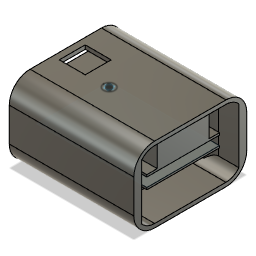
20201123 v1 (Autodesk Fusion 360 design; units mm, degrees)
Autodesk Fusion 360 part; units mm, degrees
note: some values were not read from the file. Chosen so that the rebuilt part matches the saved one: which bodies a step acts on; which face or edge a step refers to.
sketch "Sketch1" plane through (0, 0, 0) normal (0, 1, 0) x (1, 0, 0)
  line L0 (-42.5, 28) -> (42.5, 28)
  line L1 (42.5, 28) -> (42.5, -28)
  line L2 (42.5, -28) -> (-42.5, -28)
  line L3 (-42.5, -28) -> (-42.5, 28)
  line L4 (-42.5, 28) -> (42.5, -28) construction
  line L5 (42.5, 28) -> (-42.5, -28) construction
  line L6 (-42.5, 28) -> (-39, 28) construction
  line L7 (-39, 28) -> (-39, 24.5) construction
  line L8 (-39, 24.5) -> (-42.5, 24.5) construction
  line L9 (-42.5, 24.5) -> (-42.5, 28) construction
  line L10 (-39, 24.5) -> (19, 24.5) construction
  line L11 (19, 24.5) -> (19, -24.5) construction
  line L12 (19, -24.5) -> (-39, -24.5) construction
  line L13 (-39, -24.5) -> (-39, 24.5) construction
  circle A0 centre (-39, 24.5) radius 1.25
  circle A1 centre (19, 24.5) radius 1.25
  circle A2 centre (-39, -24.5) radius 1.25
  circle A3 centre (19, -24.5) radius 1.25
  dimension "d1" = 85
  dimension "d2" = 56
  dimension "d3" = 3.5
  dimension "d4" = 3.5
  dimension "d5" = 58
  dimension "d6" = 49
  dimension "d7" = 2.5
  dimension "d10" = 58
  dimension "d11" = -49
  constraint horizontal L0
  constraint perpendicular L0 L1
  constraint parallel L0 L2
  constraint parallel L1 L3
  constraint coincident L4 origin
  constraint coincident L5 origin
  constraint horizontal L6
  constraint vertical L7
  constraint horizontal L8
  constraint vertical L9
  constraint horizontal L10
  constraint vertical L11
  constraint horizontal L12
  constraint vertical L13
  constraint coincident L7.end L8.start
  measures "d1" distance of L1.end L2.end
  measures "d2" distance of L0.end L1.end
  measures "d3" distance of L0.start L6.end
  measures "d4" distance of L0.start L8.end
  measures "d5" distance of L7.end L10.end
  measures "d6" distance of L7.end L12.end
  measures "d7" diameter of A0
extrude "Extrude1" add sketch "Sketch1" along normal blind 1.5 makes body 1
sketch "Sketch2" plane through (0, 1.5, 0) normal (0, 1, 0) x (-1, 0, 0)
  circle A0 centre (-19, -24.5) radius 1.25
  circle A1 centre (39, 24.5) radius 1.25
  circle A2 centre (-19, 24.5) radius 1.25
  circle A3 centre (39, -24.5) radius 1.25
  line L0 (42.5, 28) -> (-42.5, 28)
  line L1 (-42.5, 28) -> (-42.5, -28)
  line L2 (-42.5, -28) -> (42.5, -28)
  line L3 (42.5, -28) -> (42.5, 28)
  line L4 (40.3568, -26.85) -> (41.7135, -24.5)
  line L5 (41.7135, -24.5) -> (40.3568, -22.15)
  line L6 (40.3568, -22.15) -> (37.6432, -22.15)
  line L7 (37.6432, -22.15) -> (36.2865, -24.5)
  line L8 (36.2865, -24.5) -> (37.6432, -26.85)
  line L9 (37.6432, -26.85) -> (40.3568, -26.85)
  circle A4 centre (39, -24.5) radius 4.25
  point P0 (39, -24.5)
  dimension "d14" = 2.35
  dimension "d15" = 8.5
  constraint coincident P0 A3.centre
  constraint concentric A3 A4
  measures "d14" distance of P0 L9
  measures "d15" diameter of A4
extrude "Extrude2" add sketch "Sketch2" along normal blind 5 separate body contours L3 A4 | L2 L3 A4 | L2 A4 picked at (36.4205, -25.9987) makes body 2
move_body "Move1" bodies 2 to x (1, 0, 0) y (0, 1, 0) z (0, 0, 1) at (0, 2, 0)
copy_body "Body->Comp1" bodies 1 removing the originals makes body 3 in component "raspberry"
copy_body "CutPasteBodies1" bodies 2 removing the originals makes body 4 in component "raspberry"
pattern_linear "R-Pattern1" count 2 spacing 58 along (1, 0, 0) count 2 spacing 49 along (0, 0, 1) of bodies 4 makes body 5 at (21.5784, 6.8333, -27.8785) makes body 6 at (-36.4216, 6.8333, 21.1215) makes body 7 at (21.5784, 6.8333, 21.1215) in component "raspberry"
copy_body "CopyPasteBodies1" bodies 3 makes body 8
move_body "Move2" bodies 8 to x (1, 0, 0) y (0, 1, 0) z (0, 0, 1) at (0, 9, 0)
move_body "Move3" bodies 8 to x (1, 0, 0) y (0, 1, 0) z (0, 0, 1) at (0, -0.5, 0)
extrude "Extrude1'" add 1 faces at (-19.3123, 0, 7.8904) along direction (0, -1, 0) blind 16 on bodies 3 bodies 3 in component "raspberry"
extrude "Extrude3" add 1 faces at (-19.3123, 10, 7.8904) along direction (0, 1, 0) blind 0.15 on bodies 8 bodies 8
extrude "Extrude4" cut 1 faces at (-19.3123, 10.15, 7.8904) along direction (0, -1, 0) blind 0.03 on bodies 8 bodies 8
sketch "Sketch3" plane through (0, 10.12, 0) normal (0, 1, 0) x (-1, 0, 0)
  circle A0 centre (-19, -24.5) radius 1.25
  circle A1 centre (39, 24.5) radius 1.25
  circle A2 centre (-19, 24.5) radius 1.25
  circle A3 centre (39, -24.5) radius 1.25
  line L0 (42.5, 28) -> (-42.5, 28)
  line L1 (-42.5, 28) -> (-42.5, -28)
  line L2 (-42.5, -28) -> (42.5, -28)
  line L3 (42.5, -28) -> (42.5, 28)
  line L4 (-42.5, 20) -> (42.5, 20)
  line L5 (42.5, 20) -> (42.5, -20)
  line L6 (42.5, -20) -> (-42.5, -20)
  line L7 (-42.5, -20) -> (-42.5, 20)
  line L8 (-42.5, 20) -> (42.5, -20) construction
  line L9 (42.5, 20) -> (-42.5, -20) construction
  dimension "d28" = 40
  constraint horizontal L4
  constraint perpendicular L4 L5
  constraint parallel L4 L6
  constraint parallel L5 L7
  constraint coincident L8 origin
  constraint coincident L9 origin
  measures "d28" distance of L4.end L5.end
extrude "Extrude5" add sketch "Sketch3" along normal blind 20 contours L1 L3 L4 L5 L6 L7 bodies 8
sketch "Sketch4" plane through (0, 3.5, 0) normal (0, -1, 0) x (1, 0, 0)
  line L0 (-37.6432, 22.15) -> (-40.3568, 22.15)
  line L1 (-40.3568, 22.15) -> (-41.7135, 24.5)
  line L2 (-41.7135, 24.5) -> (-40.3568, 26.85)
  line L3 (-40.3568, 26.85) -> (-37.6432, 26.85)
  line L4 (-37.6432, 26.85) -> (-36.2865, 24.5)
  line L5 (-36.2865, 24.5) -> (-37.6432, 22.15)
  circle A0 centre (-39, 24.5) radius 4.25
  line L6 (45, 28.5) -> (45, -28.5)
  line L7 (-45, -23.5) -> (-45, 23.5)
  line L8 (45, 37.5) -> (-45, -37.5) construction
  line L9 (-34.75, 24.5) -> (-34.75, 28.5)
  line L10 (-45, 0) -> (45, 0) construction
  line L11 (19, 37) -> (-39, 37) construction
  line L12 (-10, 37) -> (-10, -37.5) construction
  line L13 (23.25, 24.5) -> (23.25, 28.5)
  line L14 (14.75, 24.5) -> (14.75, 28.5)
  circle A1 centre (19, 24.5) radius 4.25
  circle A2 centre (-39, 24.5) radius 4.25
  line L15 (23.25, -24.5) -> (23.25, -28.5)
  line L16 (14.75, -24.5) -> (14.75, -28.5)
  circle A3 centre (19, -24.5) radius 4.25
  line L17 (-34.75, -24.5) -> (-34.75, -28.5)
  circle A4 centre (-39, -24.5) radius 4.25
  line L18 (48, -40.5) -> (-48, -40.5)
  line L19 (-48, -40.5) -> (-48, 40.5)
  line L20 (-48, 40.5) -> (48, 40.5)
  line L21 (48, 40.5) -> (48, -40.5)
  line L22 (32.25, 37.5) -> (36, 37.5)
  line L23 (-45, 37.5) -> (-10, 8.3333) construction
  line L24 (0, 0) -> (45, -37.5) construction
  line L25 (-25.75, 37.5) -> (5.75, 37.5)
  line L26 (36, -37.5) -> (32.25, -37.5)
  line L27 (5.75, -37.5) -> (-25.75, -37.5)
  line L28 (-43.25, -24.5) -> (-44, -24.5)
  line L29 (-43.25, 24.5) -> (-44, 24.5)
  arc A5 (5.75, -37.5) -> (14.75, -28.5) centre (5.75, -28.5) ccw
  arc A6 (23.25, -28.5) -> (32.25, -37.5) centre (32.25, -28.5) ccw
  arc A7 (32.25, 37.5) -> (23.25, 28.5) centre (32.25, 28.5) ccw
  arc A8 (14.75, 28.5) -> (5.75, 37.5) centre (5.75, 28.5) ccw
  arc A9 (-25.75, 37.5) -> (-34.75, 28.5) centre (-25.75, 28.5) ccw
  arc A10 (-34.75, -28.5) -> (-25.75, -37.5) centre (-25.75, -28.5) ccw
  arc A11 (36, -37.5) -> (45, -28.5) centre (36, -28.5) ccw
  arc A12 (45, 28.5) -> (36, 37.5) centre (36, 28.5) ccw
  arc A13 (-44, 24.5) -> (-45, 23.5) centre (-44, 23.5) ccw
  arc A14 (-45, -23.5) -> (-44, -24.5) centre (-44, -23.5) ccw
  dimension "d31" = 90
  dimension "d32" = 75
  dimension "d34" = 9
  dimension "d35" = 1
  constraint parallel L6 L7
  constraint coincident L24.start L23
  constraint coincident L8 L24.start
  constraint coincident L24.start origin
  constraint coincident A0 L29.start
  constraint coincident A0 L9.start
  constraint tangent A0 L9
  constraint parallel L3 L11
  constraint midpoint L11 L12.start
  constraint coincident L12.end L26
  constraint perpendicular L12 L26
  constraint symmetric L29.start L12 L13.start
  constraint symmetric L9.start L12 L14.start
  constraint coincident L14.start A1
  constraint tangent L14 A1
  constraint coincident L13.start A1
  constraint coincident L29.start A2
  constraint coincident L9.start A2
  constraint symmetric L29.start L10 L28.start
  constraint symmetric L9.start L10 L17.start
  constraint symmetric L10 L13.start L15.start
  constraint symmetric L10 L14.start L16.start
  constraint symmetric L10 A1 A3
  constraint symmetric L10 A2 A4
  constraint parallel L18 L26
  constraint parallel L7 L19
  constraint parallel L6 L21
  constraint coincident L12 L23.end
  constraint collinear L23 L24
  constraint collinear L26 L27
  constraint perpendicular L7 L29
  constraint coincident L7 L10.start
  constraint tangent L16 A5
  constraint tangent L27 A5
  constraint tangent L15 A6
  constraint tangent L26 A6
  constraint equal A5 A6
  constraint tangent L13 A7
  constraint tangent L22 A7
  constraint equal A5 A7
  constraint tangent L14 A8
  constraint tangent L25 A8
  constraint equal A5 A8
  constraint tangent L9 A9
  constraint tangent L25 A9
  constraint equal A5 A9
  constraint tangent L17 A10
  constraint tangent L27 A10
  constraint equal A5 A10
  constraint coincident L6 L10.end
  constraint coincident L24.end L26
  constraint coincident L24.end L6
  constraint tangent L26 A11
  constraint tangent L6 A11
  constraint equal A5 A11
  constraint coincident L8.start L6
  constraint coincident L8.start L22
  constraint tangent L6 A12
  constraint tangent L22 A12
  constraint equal A5 A12
  constraint tangent L29 A13
  constraint tangent L7 A13
  constraint tangent L28 A14
  constraint tangent L7 A14
  constraint equal A13 A14
  measures "d31" distance of L24.end L8.end
  measures "d32" distance of L8.start L24.end
  measures "d34" radius of A5
  measures "d35" radius of A13
extrude "Extrude2'" add sketch "Sketch4" against normal blind 5 contours L18 L19 L20 L21 bodies 4 5 6 7 in component "raspberry"
copy_body "CutPasteBodies2" bodies 8 removing the originals makes body 9 in component "raspberry"
copy_body "CopyPasteBodies2" bodies 4 makes body 10
move_body "Move4" bodies 10 to x (1, 0, 0) y (0, 1, 0) z (0, 0, 1) at (0, 6.5, 0)
move_body "Move5" bodies 10 to x (1, 0, 0) y (0, 1, 0) z (0, 0, 1) at (0, 10, 0)
move_body "Move6" bodies 10 to x (1, 0, 0) y (0, 1, 0) z (0, 0, 1) at (0, -9.88, 0)
extrude "Extrude6" cut 1 faces at (-40.7645, 15.12, -33.1962) along direction (0, -1, 0) blind 2 on bodies 10 bodies 10
sketch "Sketch5" plane through (0, 8.5, 0) normal (0, 1, 0) x (-1, 0, 0)
  line L0 (-17.6432, 22.15) -> (-20.3568, 22.15)
  line L1 (-20.3568, 22.15) -> (-21.7135, 24.5)
  line L2 (-21.7135, 24.5) -> (-20.3568, 26.85)
  line L3 (-20.3568, 26.85) -> (-17.6432, 26.85)
  line L4 (-17.6432, 26.85) -> (-16.2865, 24.5)
  line L5 (-16.2865, 24.5) -> (-17.6432, 22.15)
  line L6 (40.3568, 22.15) -> (37.6432, 22.15)
  line L7 (37.6432, 22.15) -> (36.2865, 24.5)
  line L8 (36.2865, 24.5) -> (37.6432, 26.85)
  line L9 (37.6432, 26.85) -> (40.3568, 26.85)
  line L10 (40.3568, 26.85) -> (41.7135, 24.5)
  line L11 (41.7135, 24.5) -> (40.3568, 22.15)
  line L12 (-17.6432, -26.85) -> (-20.3568, -26.85)
  line L13 (-20.3568, -26.85) -> (-21.7135, -24.5)
  line L14 (-21.7135, -24.5) -> (-20.3568, -22.15)
  line L15 (-20.3568, -22.15) -> (-17.6432, -22.15)
  line L16 (-17.6432, -22.15) -> (-16.2865, -24.5)
  line L17 (-16.2865, -24.5) -> (-17.6432, -26.85)
  line L18 (48, 40.5) -> (-48, 40.5)
  line L19 (-48, 40.5) -> (-48, -40.5)
  line L20 (-48, -40.5) -> (48, -40.5)
  line L21 (48, -40.5) -> (48, 40.5)
  line L22 (40.3568, -26.85) -> (37.6432, -26.85)
  line L23 (37.6432, -26.85) -> (36.2865, -24.5)
  line L24 (36.2865, -24.5) -> (37.6432, -22.15)
  line L25 (37.6432, -22.15) -> (40.3568, -22.15)
  line L26 (40.3568, -22.15) -> (41.7135, -24.5)
  line L27 (41.7135, -24.5) -> (40.3568, -26.85)
  arc A0 (43.25, -24.5) -> (34.75, -24.5) centre (39, -24.5) ccw
  line L28 (34.75, -24.5) -> (34.75, -28.5)
  arc A1 (25.75, -37.5) -> (34.75, -28.5) centre (25.75, -28.5) ccw
  line L29 (25.75, -37.5) -> (-5.75, -37.5)
  arc A2 (-14.75, -28.5) -> (-5.75, -37.5) centre (-5.75, -28.5) ccw
  line L30 (-14.75, -28.5) -> (-14.75, -24.5)
  arc A3 (-14.75, -24.5) -> (-23.25, -24.5) centre (-19, -24.5) ccw
  line L31 (-23.25, -24.5) -> (-23.25, -28.5)
  arc A4 (-32.25, -37.5) -> (-23.25, -28.5) centre (-32.25, -28.5) ccw
  line L32 (-32.25, -37.5) -> (-36, -37.5)
  arc A5 (-45, -28.5) -> (-36, -37.5) centre (-36, -28.5) ccw
  line L33 (-45, -28.5) -> (-45, 28.5)
  arc A6 (-36, 37.5) -> (-45, 28.5) centre (-36, 28.5) ccw
  line L34 (-36, 37.5) -> (-32.25, 37.5)
  arc A7 (-23.25, 28.5) -> (-32.25, 37.5) centre (-32.25, 28.5) ccw
  line L35 (-23.25, 28.5) -> (-23.25, 24.5)
  arc A8 (-23.25, 24.5) -> (-14.75, 24.5) centre (-19, 24.5) ccw
  line L36 (-14.75, 24.5) -> (-14.75, 28.5)
  arc A9 (-5.75, 37.5) -> (-14.75, 28.5) centre (-5.75, 28.5) ccw
  line L37 (-5.75, 37.5) -> (25.75, 37.5)
  arc A10 (34.75, 28.5) -> (25.75, 37.5) centre (25.75, 28.5) ccw
  line L38 (34.75, 28.5) -> (34.75, 24.5)
  arc A11 (34.75, 24.5) -> (43.25, 24.5) centre (39, 24.5) ccw
  line L39 (43.25, 24.5) -> (44, 24.5)
  arc A12 (45, 23.5) -> (44, 24.5) centre (44, 23.5) ccw
  line L40 (45, 23.5) -> (45, -23.5)
  arc A13 (44, -24.5) -> (45, -23.5) centre (44, -23.5) ccw
  line L41 (44, -24.5) -> (43.25, -24.5)
  line L42 (-19, 24.5) -> (-19, 28.25) construction
  line L43 (39, 24.5) -> (39, 28.25) construction
  arc A14 (48, 36.4333) -> (43.25, 28.5) centre (52.25, 28.5) ccw construction
  line L44 (43.25, 28.5) -> (43.25, 24.5)
  arc A15 (48, 36.4333) -> (43.25, 28.5) centre (52.25, 28.5) ccw
  line L45 (-36, 37.5) -> (-48, 37.5)
  line L46 (48, 28.25) -> (-48, 28.25) construction
  line L47 (-48, 28.25) -> (-48, -28.25) construction
  line L48 (-48, -28.25) -> (48, -28.25) construction
  line L49 (48, -28.25) -> (48, 28.25) construction
  line L50 (48, 28.25) -> (-48, -28.25) construction
  line L51 (-48, 28.25) -> (48, -28.25) construction
  line L52 (-48, 28.25) -> (48, 28.25)
  line L53 (48, -28.25) -> (-48, -28.25)
  line L54 (-48, 0) -> (48, 0) construction
  arc A16 (43.25, -28.5) -> (48, -36.4333) centre (52.25, -28.5) ccw construction
  arc A17 (43.25, -28.5) -> (48, -36.4333) centre (52.25, -28.5) ccw
  line L55 (43.25, -28.5) -> (43.25, -24.5)
  line L56 (-36, -37.5) -> (-48, -37.5)
  dimension "d40" = 3.75
  dimension "d41" = 3.75
  dimension "d42" = 9
  constraint coincident A8.centre L42.start
  constraint vertical L42
  constraint coincident A11.centre L43.start
  constraint parallel L38 L43
  constraint coincident A11.end L39.start
  constraint concentric A14 A15
  constraint coincident L21 A14.start
  constraint coincident A6.start L34.start
  constraint coincident L19 L45.end
  constraint tangent A6 L45
  constraint horizontal L46
  constraint perpendicular L46 L47
  constraint parallel L46 L48
  constraint parallel L47 L49
  constraint coincident L21 L46.start
  constraint coincident L50 origin
  constraint coincident L51 origin
  constraint midpoint L19 L54.start
  constraint midpoint L21 L54.end
  constraint symmetric A11.end L54 A0.start
  constraint symmetric A14.end L54 A16.start
  constraint symmetric A14 L54 A16
  constraint symmetric A15 L54 A17
  constraint symmetric A14.start L54 A16.end
  constraint coincident L32.end A5.end
  constraint coincident L19 L56.end
  constraint tangent A5 L56
  measures "d40" distance of A8.centre L42.end
  measures "d41" distance of A11.centre L43.end
  measures "d42" radius of A14
extrude "Extrude3'" cut sketch "Sketch5" against normal blind 25 contours L21 L44 A15 L52 | L19 L33 A6 L45 L52 | L21 L39 A12 L40 A13 L41 L44 L52 L53 L55 | L19 L33 L52 L53 | L21 L53 A17 L55 | L19 A5 L33 L53 L56 bodies 4 makes body 11 at (-41.9239, 8.5, 36.3378) in component "raspberry"
extrude "Extrude7" add sketch "Sketch5" along normal blind 2 contours L19 L20 L21 L28 A1 L29 A2 L30 L31 A4 L32 L53 A17 L55 L56 bodies 10
extrude "Extrude8" add sketch "Sketch5" along normal blind 3 contours L18 L19 L21 L34 A7 L35 L36 A9 L37 A10 L38 L44 A15 L45 L52 bodies 10
extrude "Extrude9" cut sketch "Sketch5" along normal blind 20 contours L21 L44 A15 L52 | L19 L33 A6 L45 L52 | L21 L39 A12 L40 A13 L41 L44 L52 L53 L55 | L19 L33 L52 L53 | L21 L53 A17 L55 | L19 A5 L33 L53 L56 bodies 10 makes body 12 at (-41.9239, 13.12, 36.3378)
combine "Combine1" operation add target body 10 tool bodies 4
combine "Combine2" operation add target body 12 tool bodies 11
copy_body "CutPasteBodies3" bodies 12 removing the originals makes body 13 in component "raspberry"
copy_body "CutPasteBodies4" bodies 10 removing the originals makes body 14 in component "raspberry"
sketch "Sketch6" plane through (0, 13.12, 0) normal (0, 1, 0) x (-1, 0, 0)
  line L0 (40.3568, -26.85) -> (37.6432, -26.85)
  line L1 (37.6432, -26.85) -> (36.2865, -24.5)
  line L2 (36.2865, -24.5) -> (37.6432, -22.15)
  line L3 (37.6432, -22.15) -> (40.3568, -22.15)
  line L4 (40.3568, -22.15) -> (41.7135, -24.5)
  line L5 (41.7135, -24.5) -> (40.3568, -26.85)
  line L6 (-17.6432, -26.85) -> (-20.3568, -26.85)
  line L7 (-20.3568, -26.85) -> (-21.7135, -24.5)
  line L8 (-21.7135, -24.5) -> (-20.3568, -22.15)
  line L9 (-20.3568, -22.15) -> (-17.6432, -22.15)
  line L10 (-17.6432, -22.15) -> (-16.2865, -24.5)
  line L11 (-16.2865, -24.5) -> (-17.6432, -26.85)
  line L12 (-32.25, -37.5) -> (-48, -37.5)
  line L13 (-48, -37.5) -> (-48, -40.5)
  line L14 (-48, -40.5) -> (48, -40.5)
  line L15 (48, -40.5) -> (48, -36.4333)
  arc A0 (43.25, -28.5) -> (48, -36.4333) centre (52.25, -28.5) ccw
  line L16 (43.25, -28.5) -> (43.25, -24.5)
  arc A1 (43.25, -24.5) -> (34.75, -24.5) centre (39, -24.5) ccw
  line L17 (34.75, -24.5) -> (34.75, -28.5)
  arc A2 (25.75, -37.5) -> (34.75, -28.5) centre (25.75, -28.5) ccw
  line L18 (25.75, -37.5) -> (-5.75, -37.5)
  arc A3 (-14.75, -28.5) -> (-5.75, -37.5) centre (-5.75, -28.5) ccw
  line L19 (-14.75, -28.5) -> (-14.75, -24.5)
  arc A4 (-14.75, -24.5) -> (-23.25, -24.5) centre (-19, -24.5) ccw
  line L20 (-23.25, -24.5) -> (-23.25, -28.5)
  arc A5 (-32.25, -37.5) -> (-23.25, -28.5) centre (-32.25, -28.5) ccw
  circle A6 centre (-19, -24.5) radius 1.375
  circle A7 centre (-19, -24.5) radius 2.7135
  circle A8 centre (39, -24.5) radius 2.7135
  circle A9 centre (39, -24.5) radius 1.375
  circle A10 centre (-19, 24.5) radius 2.7135
  circle A11 centre (-19, 24.5) radius 1.375
  circle A12 centre (39, 24.5) radius 2.7135
  circle A13 centre (39, 24.5) radius 1.375
  dimension "d51" = 2.75
  dimension "d54" = 58
  dimension "d55" = 49
  constraint concentric A4 A6
  constraint concentric A6 A7
  constraint coincident L6.start A7
  measures "d51" diameter of A6
extrude "Extrude5'" add sketch "Sketch6" against normal blind 3 contours L0 L1 L2 L3 L4 L5 | L6 L7 L8 L9 L10 L11 | A10 | A12 bodies 13 14 in component "raspberry"
extrude "Extrude4'" cut sketch "Sketch6" against normal blind 3 contours L0 L1 L2 L3 L4 L5 | L6 L7 L8 L9 L10 L11 | A10 | A12 bodies 13 in component "raspberry"
extrude "Extrude6'" add sketch "Sketch6" against normal blind 3 contours A10 | A12 bodies 13 in component "raspberry"
extrude "Extrude7'" cut 1 faces at (-19.3123, -16, 7.8904) along direction (0, 1, 0) blind 16 on bodies 3 bodies 3 in component "raspberry"
extrude "Extrude10" add sketch "Sketch2" along normal blind 7 separate body contours L4 L5 L6 L7 L8 L9 makes body 15
copy_body "CopyPasteBodies3" bodies 15 makes body 16
move_body "Move7" bodies 16 to x (1, 0, 0) y (0, 1, 0) z (0, 0, 1) at (0, -18, 0)
move_body "Move8" bodies 16 to x (1, 0, 0) y (0, 1, 0) z (0, 0, 1) at (0, 9.5, 0)
pattern_linear "R-Pattern1'" count 2 spacing 49 along (0, 0, 1) count 2 spacing 58 along (1, 0, 0) of bodies 16 15 makes body 17 at (-40.2438, 6.1667, 24.3755) makes body 18 at (17.7562, 6.1667, -24.6245) makes body 19 at (17.7562, 6.1667, 24.3755) makes body 20 at (-40.2438, -2.3333, 24.3755) makes body 21 at (17.7562, -2.3333, -24.6245) makes body 22 at (17.7562, -2.3333, 24.3755)
copy_body "CopyPasteBodies4" bodies 3 makes body 23
move_body "Move9" bodies 23 to x (1, 0, 0) y (0, 1, 0) z (0, 0, 1) at (0, -40, 0)
move_body "Move10" bodies 23 to x (1, 0, 0) y (0, 1, 0) z (0, 0, 1) at (0, 31.5, 0)
extrude "Extrude11" cut 1 faces at (42.5, -8, -9.3333) along direction (-1, 0, 0) blind 19 on bodies 23 bodies 23
extrude "Extrude12" add 1 faces at (-19.3612, -8.5, 7.8833) along direction (0, -1, 0) blind 8.6 on bodies 23 bodies 23
sketch "Sketch7" plane through (-48, 0, 0) normal (-1, 0, 0) x (0, 0, 1)
  line L0 (-36.4333, 3.5) -> (-36.4333, 13.12)
  line L1 (-36.4333, 13.12) -> (-40.5, 13.12)
  line L2 (-40.5, 13.12) -> (-40.5, 3.5)
  line L3 (-40.5, 3.5) -> (-36.4333, 3.5)
  line L4 (-27.5, 32) -> (27.5, 32)
  line L5 (40.5, 19) -> (40.5, -7)
  line L6 (27.5, -20) -> (-27.5, -20)
  line L7 (-40.5, -7) -> (-40.5, 19)
  line L8 (-40.5, 32) -> (40.5, -20) construction
  line L9 (40.5, 32) -> (-40.5, -20) construction
  arc A0 (-27.5, 32) -> (-40.5, 19) centre (-27.5, 19) ccw
  arc A1 (-40.5, -7) -> (-27.5, -20) centre (-27.5, -7) ccw
  arc A2 (27.5, -20) -> (40.5, -7) centre (27.5, -7) ccw
  arc A3 (40.5, 19) -> (27.5, 32) centre (27.5, 19) ccw
  arc A4 (43.5, 19) -> (27.5, 35) centre (27.5, 19) ccw
  line L10 (-27.5, 35) -> (27.5, 35)
  arc A5 (-27.5, 35) -> (-43.5, 19) centre (-27.5, 19) ccw
  line L11 (-43.5, -7) -> (-43.5, 19)
  arc A6 (-43.5, -7) -> (-27.5, -23) centre (-27.5, -7) ccw
  line L12 (27.5, -23) -> (-27.5, -23)
  arc A7 (27.5, -23) -> (43.5, -7) centre (27.5, -7) ccw
  line L13 (43.5, 19) -> (43.5, -7)
  point P0 (0, 6)
  dimension "d74" = 52
  dimension "d75" = 13
  dimension "d76" = -3
  constraint horizontal L4
  constraint perpendicular L4 L5
  constraint parallel L4 L6
  constraint parallel L5 L7
  constraint coincident L8 P0
  constraint coincident L9 P0
  constraint coincident L8.start L4
  constraint coincident L8.start L7
  constraint tangent L4 A0
  constraint tangent L7 A0
  constraint coincident L9.end L7
  constraint coincident L9.end L6
  constraint tangent L7 A1
  constraint tangent L6 A1
  constraint equal A0 A1
  constraint coincident L8.end L6
  constraint coincident L8.end L5
  constraint tangent L6 A2
  constraint tangent L5 A2
  constraint equal A0 A2
  constraint coincident L9.start L5
  constraint coincident L9.start L4
  constraint tangent L5 A3
  constraint tangent L4 A3
  constraint equal A0 A3
  measures "d74" distance of L9.start L8.end
  measures "d75" radius of A0
extrude "Extrude8'" add sketch "Sketch7" against normal blind 96 bodies 13 14 in component "raspberry"
sketch "Sketch8" plane through (0, 13.12, 0) normal (0, 1, 0) x (-1, 0, 0)
  circle A0 centre (-19, -24.5) radius 1.375
  circle A1 centre (39, -24.5) radius 1.375
  line L0 (-32.25, -37.5) -> (-48, -37.5)
  line L1 (-48, -37.5) -> (-48, -40.5)
  line L2 (-48, -40.5) -> (48, -40.5)
  line L3 (48, -40.5) -> (48, -36.4333)
  arc A2 (43.25, -28.5) -> (48, -36.4333) centre (52.25, -28.5) ccw
  line L4 (43.25, -28.5) -> (43.25, -24.5)
  arc A3 (43.25, -24.5) -> (34.75, -24.5) centre (39, -24.5) ccw
  line L5 (34.75, -24.5) -> (34.75, -28.5)
  arc A4 (25.75, -37.5) -> (34.75, -28.5) centre (25.75, -28.5) ccw
  line L6 (25.75, -37.5) -> (-5.75, -37.5)
  arc A5 (-14.75, -28.5) -> (-5.75, -37.5) centre (-5.75, -28.5) ccw
  line L7 (-14.75, -28.5) -> (-14.75, -24.5)
  arc A6 (-14.75, -24.5) -> (-23.25, -24.5) centre (-19, -24.5) ccw
  line L8 (-23.25, -24.5) -> (-23.25, -28.5)
  arc A7 (-32.25, -37.5) -> (-23.25, -28.5) centre (-32.25, -28.5) ccw
  line L9 (-23.25, -28.5) -> (-14.75, -28.5)
  line L10 (34.75, -28.5) -> (43.25, -28.5)
  line L11 (48, 0) -> (-48, 0) construction
  line L12 (-23.25, 28.5) -> (-14.75, 28.5)
  line L13 (34.75, 28.5) -> (43.25, 28.5)
  constraint coincident L8.end A7.end
  constraint coincident A5.start L7.start
  constraint coincident L5.end A4.end
  constraint coincident A2.start L4.start
  constraint horizontal L11
  constraint symmetric L8.end L11 L12.start
  constraint symmetric A5.start L11 L12.end
  constraint symmetric L5.end L11 L13.start
  constraint symmetric A2.start L11 L13.end
extrude "Extrude13" add sketch "Sketch8" along normal blind 24 separate body contours L0 L1 L2 L3 A2 A4 L6 A5 A7 L9 L10 makes body 24
copy_body "CopyPasteBodies5" bodies 24 makes body 25
move_body "Move11" bodies 24 to x (1, 0, 0) y (0, 1, 0) z (0, 0, 1) at (0, -24, 64.875)
move_body "Move12" bodies 24 to x (1, 0, 0) y (0, -1, 0) z (0, 0, -1) at (0, -21.76, 48.75)
move_body "Move13" bodies 24 to x (1, 0, 0) y (0, 1, 0) z (0, 0, 1) at (0, 48, 12)
move_body "Move14" bodies 24 to x (1, 0, 0) y (0, 1, 0) z (0, 0, 1) at (0, 0, 11)
move_body "Move15" bodies 24 to x (1, 0, 0) y (0, 1, 0) z (0, 0, 1) at (0, 0, -6.875)
copy_body "CopyPasteBodies6" bodies 25 24 makes body 26 makes body 27
move_body "Move16" bodies 26 27 to x (1, 0, 0) y (0, 1, 0) z (0, 0, 1) at (0, -65, 0)
move_body "Move17" bodies 26 27 to x (1, 0, 0) y (0, 1, 0) z (0, 0, 1) at (0, 31.38, 0)
move_face "OffsetFaces1" offset -5 2 faces at (20.4167, 29.12, -28.5) (-40.4167, 29.12, -28.5) on bodies 25
move_face "OffsetFaces2" offset -5 6 faces at (20.4167, 21.12, 28.5) (-40.4167, 21.12, 28.5) (20.4167, -4.5, -28.5) (-40.4167, -4.5, -28.5) (20.4167, -12.5, 28.5) (-40.4167, -4.5, 28.5) on bodies 24 26 27
combine "Combine3" operation add target body 25 tool bodies 13 26 27 24
sketch "Sketch9" plane through (-48, 0, 0) normal (-1, 0, 0) x (0, 0, 1)
  arc A0 (36.4333, 32.2739) -> (27.5, 35) centre (27.5, 19) ccw
  line L0 (27.5, 35) -> (-27.5, 35)
  arc A1 (-27.5, 35) -> (-36.4333, 32.2739) centre (-27.5, 19) ccw
  line L1 (-36.4333, 32.2739) -> (-36.4333, 37.12)
  line L2 (-36.4333, 37.12) -> (-40.5, 37.12)
  line L3 (-40.5, 37.12) -> (-40.5, 28.3274)
  arc A2 (-40.5, 28.3274) -> (-43.5, 19) centre (-27.5, 19) ccw
  line L4 (-43.5, 19) -> (-43.5, -7)
  arc A3 (-43.5, -7) -> (-40.5, -16.3274) centre (-27.5, -7) ccw
  line L5 (-40.5, -16.3274) -> (-40.5, -20.5)
  line L6 (-40.5, -20.5) -> (-36.4333, -20.5)
  line L7 (-36.4333, -20.5) -> (-36.4333, -20.2739)
  arc A4 (-36.4333, -20.2739) -> (-27.5, -23) centre (-27.5, -7) ccw
  line L8 (-27.5, -23) -> (27.5, -23)
  arc A5 (27.5, -23) -> (36.4333, -20.2739) centre (27.5, -7) ccw
  line L9 (36.4333, -20.2739) -> (36.4333, -20.5)
  line L10 (36.4333, -20.5) -> (40.5, -20.5)
  line L11 (40.5, -20.5) -> (40.5, -16.3274)
  arc A6 (40.5, -16.3274) -> (43.5, -7) centre (27.5, -7) ccw
  line L12 (43.5, -7) -> (43.5, 19)
  arc A7 (43.5, 19) -> (40.5, 28.3274) centre (27.5, 19) ccw
  line L13 (40.5, 28.3274) -> (40.5, 37.12)
  line L14 (40.5, 37.12) -> (36.4333, 37.12)
  line L15 (36.4333, 37.12) -> (36.4333, 32.2739)
  line L16 (36.4333, 28.4444) -> (36.4333, -16.4444)
  arc A8 (27.5, -20) -> (36.4333, -16.4444) centre (27.5, -7) ccw
  line L17 (27.5, -20) -> (-27.5, -20)
  arc A9 (-36.4333, -16.4444) -> (-27.5, -20) centre (-27.5, -7) ccw
  line L18 (-36.4333, -16.4444) -> (-36.4333, 28.4444)
  arc A10 (-27.5, 32) -> (-36.4333, 28.4444) centre (-27.5, 19) ccw
  line L19 (-27.5, 32) -> (27.5, 32)
  arc A11 (36.4333, 28.4444) -> (27.5, 32) centre (27.5, 19) ccw
  arc A12 (-27.5, 35) -> (-43.5, 19) centre (-27.5, 19) ccw
  arc A13 (-43.5, -7) -> (-27.5, -23) centre (-27.5, -7) ccw
  arc A14 (43.5, 19) -> (27.5, 35) centre (27.5, 19) ccw
  arc A15 (36.4333, -20.2739) -> (43.5, -7) centre (27.5, -7) ccw
  line L20 (-50, 44) -> (56, 44)
  line L21 (56, 44) -> (56, -36)
  line L22 (56, -36) -> (-50, -36)
  line L23 (-50, -36) -> (-50, 44)
  line L24 (-43.5, 35) -> (43.5, 35)
  line L25 (43.5, 35) -> (43.5, -23.0093)
  line L26 (43.5, -23.0093) -> (-43.5, -23.0093)
  line L27 (-43.5, -23.0093) -> (-43.5, 35)
  constraint concentric A1 A12
  constraint coincident A1.end A12
  constraint concentric A5 A15
  constraint concentric A3 A13
  constraint horizontal L20
  constraint vertical L21
  constraint horizontal L22
  constraint vertical L23
  constraint horizontal L24
  constraint vertical L25
  constraint horizontal L26
  constraint vertical L27
extrude "Extrude14" cut sketch "Sketch9" against normal blind 120 contours A0 L15 A14 L24 | L13 L15 A14 L24 | L13 L14 L15 L24 | A7 L13 A14 L24 L25 | A1 L1 A12 L24 | L1 L3 A12 L24 | L1 L2 L3 L24 | A3 L5 L6 L7 A4 L8 A5 L9 L10 L11 A6 A13 A15 L25 L26 L27 | L3 A2 A12 L24 L27 | L9 L10 L11 A15 | L5 L6 L7 A13 | L20 L21 L22 L23 bodies 25
copy_body "CutPasteBodies5" bodies 15 16 17 18 19 20 21 22 removing the originals makes body 28 makes body 29 makes body 30 makes body 31 makes body 32 makes body 33 makes body 34 makes body 35 in component "raspberry"
copy_body "CutPasteBodies6" bodies 23 removing the originals makes body 36 in component "raspberry"
copy_body "CutPasteBodies7" bodies 25 removing the originals makes body 37 in component "raspberry"
sketch "Sketch10" plane through (0, 0, -28) normal (0, 0, -1) x (-1, 0, 0)
  line L0 (42.5, 10.12) -> (-42.5, 10.12)
  line L1 (-42.5, 10.12) -> (-42.5, 8.5)
  line L2 (-42.5, 8.5) -> (42.5, 8.5)
  line L3 (42.5, 8.5) -> (42.5, 10.12)
  line L4 (39, 9) -> (24.9, 9) construction
  circle A0 centre (24.9, 9) radius 5
  dimension "d85" = 14.1
  dimension "d86" = 10
  constraint perpendicular L3 L4
  constraint coincident L4.end A0.centre
  measures "d85" distance of L4.start L4.end
  measures "d86" diameter of A0
extrude "Extrude9'" cut sketch "Sketch10" along normal blind 18 contours L0 L2 A0 | L2 A0 bodies 37 in component "raspberry"
fillet "Fillet1" radius 3.5 2 edges at (-24.9, 4, -43.5) (-24.9, 10.12, -43.5) on bodies 37 in component "raspberry"
sketch "Sketch11" plane through (0, -23, 0) normal (0, -1, 0) x (1, 0, 0)
  line L0 (-48, 27.5) -> (-48, -27.5)
  line L1 (-48, -27.5) -> (48, -27.5)
  line L2 (48, -27.5) -> (48, 27.5)
  line L3 (48, 27.5) -> (-48, 27.5)
  line L4 (-48, 0) -> (-33, 0) construction
  line L5 (-43, 10) -> (-23, 10)
  line L6 (-23, 10) -> (-23, -10)
  line L7 (-23, -10) -> (-43, -10)
  line L8 (-43, -10) -> (-43, 10)
  line L9 (-43, 10) -> (-23, -10) construction
  line L10 (-23, 10) -> (-43, -10) construction
  point P0 (-33, 0)
  dimension "d91" = 20
  constraint midpoint L0 L4.start
  constraint perpendicular L0 L4
  constraint horizontal L5
  constraint perpendicular L5 L6
  constraint parallel L5 L7
  constraint parallel L6 L8
  constraint coincident L9 P0
  constraint coincident L10 P0
  constraint coincident P0 L4.end
  measures "d91" distance of L5.end L6.end
extrude "Extrude10'" cut sketch "Sketch11" against normal blind 70 contours L5 L6 L7 L8 bodies 37 in component "raspberry"
extrude "Extrude11'" cut 2 faces at (-39.0343, 13.12, 28.5041) (19.0343, 13.12, 28.5041) along direction (0, -1, 0) blind 1 on bodies 37 bodies 37 in component "raspberry"
copy_body "CopyPasteBodies7" bodies 33 makes body 38
move_body "Move18" bodies 38 to x (1, 0, 0) y (0, 1, 0) z (0, 0, 1) at (0, 28, 0)
move_body "Move19" bodies 38 to x (1, 0, 0) y (0, 1, 0) z (0, 0, 1) at (0, -8.88, 0)
extrude "Extrude15" add 1 faces at (-37.2678, 19.12, 23.5359) along direction (0, 1, 0) blind 12.88 on bodies 38 bodies 38
extrude "Extrude12'" cut 2 faces at (-39.0343, 13.12, -28.5041) (19.0343, 13.12, -28.5041) along direction (0, -1, 0) blind 1 on bodies 37 bodies 37 in component "raspberry"
pattern_linear "R-Pattern2" count 2 spacing 49 along (0, 0, -1) count 2 spacing 58 along (1, 0, 0) of bodies 38 makes body 39 at (-40.2438, 25.3733, -24.6245) makes body 40 at (17.7562, 25.3733, 24.3755) makes body 41 at (17.7562, 25.3733, -24.6245)
component "raspberry" placed x (1, 0, 0) y (0, 1, 0) z (0, 0, 1) at (0, 0, 0)
equation "d14 = ( 4.7 / 2 ) * 1 mm"
equation "d62 = -17.50 mm + 1.5 mm"
named bodies: "raspberry", "support bolt", "frame board", "support bolt (1)", "support bolt (2)", "support bolt (3)", "battery board", "frame board (1)", "bolt", "bolt (1)", "bolt (2)", "bolt (3)", "bolt (4)", "bolt (1) (1)", "bolt (1) (2)", "bolt (1) (3)", "raspberry (1)", "servo board", "frame", "bolt (1) (1) (1)", "bolt (1) (1) (2)", "bolt (1) (1) (3)"
